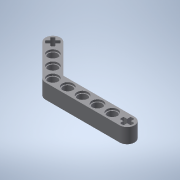
# Autodesk Inventor part: 9M Beam A 4X6
Saved by Autodesk Inventor 2021 (Build 250183000, 183)
## iProperties
Created: 2014-02-17
Part Number: 9M Beam A 4X6
Document SubType Name: Modeling
Designer: jleonard
Density: 1 g/cm^3
Material: Generic
Appearance: Default
Author: jleonard
Autodesk Inventor part; units mm, degrees
ref_plane "YZ Plane" through (0, 0, 0) normal (1, 0, 0) x (0, 1, 0)
ref_plane "XZ Plane" through (0, 0, 0) normal (0, 1, 0) x (-1, 0, 0)
ref_plane "XY Plane" through (0, 0, 0) normal (0, 0, 1) x (1, 0, 0)
sketch "Sketch1" plane through (0, 0, 0) normal (0, 0, 1) x (1, 0, 0)
  arc A0 (-54.1421, 19.799) -> (-59.799, 14.1421) centre (-56.9706, 16.9706) ccw
  arc A1 (0, -4) -> (0, 4) centre (0, 0) ccw
  line L0 (-42.8284, -2.8284) -> (-59.799, 14.1421)
  line L1 (-38.3431, 4) -> (-54.1421, 19.799)
  line L2 (-75.9529, 0) -> (17.3255, 0) projected
  line L3 (0, -9.663) -> (0, 28.0092) projected
  line L4 (0, -4) -> (-40, -4)
  line L5 (0, 4) -> (-38.3431, 4)
  arc A2 (-42.8284, -2.8284) -> (-40, -4) centre (-40, 0) ccw
  dimension "d13" = 4
  dimension "d15" = 0
  dimension "d16" = 0
  dimension "d25" = 4
  dimension "d27" = 135
  dimension "d29" = 40
  dimension "d35" = 135
  dimension "d36" = 4
  dimension "d37" = 24
  dimension "d142" = 24
  constraints: 8 end point, 6 point on circle, 4 tangent, 3 centre point, 1 parallel, 1 perpendicular, 1 point on line
  measures "d13" radius of A1
  measures "d15" distance from line of L3 A1.centre
  measures "d16" distance from line of L2 A1.centre
  measures "d25" radius of A0
  measures "d27" angle of L0 L4
  measures "d29" distance of L4.start L4.end
  measures "d35" angle of L5 L1
  measures "d36" radius of A2
  measures "d37" distance of A2.centre A0.centre
  measures "d142" distance of L0.start L0.end
extrude "Extrusion1" add sketch "Sketch1" along normal blind 8
sketch "Sketch2" plane through (0, 0, 8) normal (0, 0, 1) x (1, 0, 0)
  arc A0 (-54.1421, 19.799) -> (-59.799, 14.1421) centre (-56.9706, 16.9706) ccw projected
  line L0 (-42.8284, -2.8284) -> (-59.799, 14.1421) projected
  arc A1 (-58.2635, 19.6777) -> (-59.6777, 18.2635) centre (-56.9706, 16.9706) ccw
  arc A2 (-59.6777, 15.6777) -> (-58.2635, 14.2635) centre (-56.9706, 16.9706) ccw
  arc A3 (-55.6777, 14.2635) -> (-54.2635, 15.6777) centre (-56.9706, 16.9706) ccw
  arc A4 (-54.2635, 18.2635) -> (-55.6777, 19.6777) centre (-56.9706, 16.9706) ccw
  line L1 (-54.2635, 18.2635) -> (-55.5563, 16.9706)
  line L2 (-56.9706, 15.5563) -> (-58.2635, 14.2635)
  line L3 (-59.6777, 18.2635) -> (-58.3848, 16.9706)
  line L4 (-56.9706, 15.5563) -> (-55.6777, 14.2635)
  line L5 (-55.6777, 19.6777) -> (-56.9706, 18.3848)
  line L6 (-58.3848, 16.9706) -> (-59.6777, 15.6777)
  line L7 (-58.2635, 19.6777) -> (-56.9706, 18.3848)
  line L8 (-55.5563, 16.9706) -> (-54.2635, 15.6777)
  dimension "d46" = 3
  dimension "d47" = 3
  dimension "d48" = 3
  dimension "d49" = 3
  dimension "d50" = 2
  dimension "d51" = 2
  dimension "d52" = 2
  dimension "d53" = 2
  dimension "d54" = 1
  dimension "d55" = 1
  dimension "d56" = 1
  dimension "d57" = 1
  dimension "d58" = 90
  dimension "d59" = 90
  dimension "d60" = 90
  dimension "d61" = 90
  constraints: 16 end point, 8 point on circle, 4 centre point, 1 coincident
  measures "d46" radius of A4
  measures "d47" radius of A1
  measures "d48" radius of A2
  measures "d49" radius of A3
  measures "d50" distance between parallel lines of L6 L2
  measures "d51" distance between parallel lines of L8 L4
  measures "d52" distance between parallel lines of L5 L1
  measures "d53" distance between parallel lines of L7 L3
  measures "d54" distance from line of L3 A0.centre
  measures "d55" distance from line of L2 A0.centre
  measures "d56" distance from line of L8 A0.centre
  measures "d57" distance from line of L5 A1.centre
  measures "d58" angle of L5 L7
  measures "d59" angle of L8 L1
  measures "d60" angle of L2 L4
  measures "d61" angle of L0 L2
extrude "Extrusion2" cut sketch "Sketch2" against normal through all
sketch "Sketch3" plane through (0, 0, 8) normal (0, 0, 1) x (1, 0, 0)
  arc A0 (0, -4) -> (0, 4) centre (0, 0) ccw projected
  arc A1 (1, 2.8284) -> (-1, 2.8284) centre (0, 0) ccw
  arc A2 (-2.8284, 1) -> (-2.8284, -1) centre (0, 0) ccw
  arc A3 (-1, -2.8284) -> (1, -2.8284) centre (0, 0) ccw
  arc A4 (2.8284, -1) -> (2.8284, 1) centre (0, 0) ccw
  line L0 (-2.8284, -1) -> (-1, -1)
  line L1 (1, -1) -> (2.8284, -1)
  line L2 (-1, -2.8284) -> (-1, -1)
  line L3 (-1, 1) -> (-1, 2.8284)
  line L4 (-2.8284, 1) -> (-1, 1)
  line L5 (1, 1) -> (2.8284, 1)
  line L6 (1, -2.8284) -> (1, -1)
  line L7 (1, 1) -> (1, 2.8284)
  dimension "d65" = 3
  dimension "d66" = 3
  dimension "d67" = 3
  dimension "d68" = 3
  dimension "d69" = 2
  dimension "d70" = 2
  dimension "d71" = 2
  dimension "d72" = 2
  dimension "d73" = 90
  dimension "d74" = 90
  dimension "d75" = 90
  dimension "d76" = 1
  dimension "d77" = 1
  dimension "d78" = 1
  dimension "d79" = 1
  dimension "d80" = 2.8284
  constraints: 16 end point, 8 point on circle, 4 centre point, 1 coincident
  measures "d65" radius of A1
  measures "d66" radius of A4
  measures "d67" radius of A3
  measures "d68" radius of A2
  measures "d69" distance between parallel lines of L0 L4
  measures "d70" distance between parallel lines of L7 L3
  measures "d71" distance between parallel lines of L1 L5
  measures "d72" distance between parallel lines of L6 L2
  measures "d73" angle of L5 L7
  measures "d74" angle of L6 L1
  measures "d75" angle of L2 L0
  measures "d76" distance from line of A0.centre L3
  measures "d77" distance from line of A1.centre L0
  measures "d78" distance from line of L6 A0.centre
  measures "d79" distance from line of L5 A0.centre
  measures "d80" vertical distance of A0.centre L3.end
extrude "Extrusion3" cut sketch "Sketch3" against normal through all
sketch "Sketch10" plane through (0, 0, 8) normal (0, 0, 1) x (1, 0, 0)
  circle A0 centre (-8, 0) radius 2.5
  line L0 (-73.9647, 0) -> (16.9941, 0) projected
  line L1 (0, -21.6115) -> (0, 28.0676) projected
  circle A1 centre (-16, 0) radius 2.5
  circle A2 centre (-24, 0) radius 2.5
  circle A3 centre (-32, 0) radius 2.5
  circle A4 centre (-40, 0) radius 2.5
  point P0 (0, 0)
  dimension "d143" = 5
  dimension "d144" = 8
  dimension "d145" = 0
  dimension "d150" = 8
  constraints: 5 centre point, 1 horizontal, 8 other
  measures "d143" diameter of A0
  measures "d144" distance from line of L1 A0.centre
  measures "d145" distance from line of L0 A0.centre
  measures "d150" distance of A0.centre A1.centre
extrude "Extrusion10" cut sketch "Sketch10" against normal through all
sketch "Sketch11" plane through (0, 0, 8) normal (0, 0, 1) x (1, 0, 0)
  circle A0 centre (-45.6569, 5.6569) radius 2.5
  line L0 (-73.9647, 0) -> (16.9941, 0) projected
  line L1 (0, -8.9941) -> (0, 25.9647) projected
  line L2 (-54.1421, 19.799) -> (-38.3431, 4) projected
  circle A1 centre (-40, 0) radius 2.5 projected
  circle A2 centre (-51.3137, 11.3137) radius 2.5
  point P0 (0, 0)
  dimension "d155" = 5
  dimension "d157" = 4
  dimension "d158" = 8
  dimension "d161" = 8
  constraints: 2 centre point, 3 other
  measures "d155" diameter of A0
  measures "d157" distance from line of L2 A0.centre
  measures "d158" distance of A1.centre A0.centre
  measures "d161" distance of A0.centre A2.centre
extrude "Extrusion11" cut sketch "Sketch11" against normal through all contours A0 | A2
sketch "Sketch12" plane through (0, 0, 8) normal (0, 0, 1) x (1, 0, 0)
  circle A0 centre (-8, 0) radius 2.5 projected
  circle A1 centre (-8, 0) radius 3
  line L0 (-73.9647, 0) -> (16.9941, 0) projected
  circle A2 centre (-16, 0) radius 3
  circle A3 centre (-24, 0) radius 3
  circle A4 centre (-32, 0) radius 3
  circle A5 centre (-40, 0) radius 3
  point P0 (0, 0)
  dimension "d168" = 6
  dimension "d171" = 8
  constraints: 5 centre point, 1 coincident, 1 horizontal, 8 other
  measures "d168" diameter of A1
  measures "d171" distance of A1.centre A2.centre
extrude "Extrusion12" cut sketch "Sketch12" against normal blind 1
sketch "Sketch13" plane through (0, 0, 8) normal (0, 0, 1) x (1, 0, 0)
  circle A0 centre (-45.6569, 5.6569) radius 2.5 projected
  circle A1 centre (-51.3137, 11.3137) radius 2.5 projected
  circle A2 centre (-51.3137, 11.3137) radius 3
  circle A3 centre (-45.6569, 5.6569) radius 3
  point P0 (0, 0)
  dimension "d178" = 6
  dimension "d179" = 6
  constraints: 2 centre point, 2 coincident
  measures "d178" diameter of A2
  measures "d179" diameter of A3
extrude "Extrusion13" cut sketch "Sketch13" against normal blind 1 contours A0 | A1 | A2 | A3
sketch "Sketch14" plane through (0, 0, 0) normal (0, 0, -1) x (-1, 0, 0)
  circle A0 centre (8, 0) radius 2.5 projected
  circle A1 centre (51.3137, 11.3137) radius 2.5 projected
  circle A2 centre (45.6569, 5.6569) radius 2.5 projected
  circle A3 centre (45.6569, 5.6569) radius 3
  circle A4 centre (51.3137, 11.3137) radius 3
  circle A5 centre (8, 0) radius 3 projected
  circle A6 centre (8, 0) radius 3
  line L0 (73.9647, 0) -> (-16.9941, 0) projected
  line L1 (0, -4) -> (40, -4) projected
  circle A7 centre (16, 0) radius 3
  circle A8 centre (24, 0) radius 3
  circle A9 centre (32, 0) radius 3
  circle A10 centre (40, 0) radius 3
  point P0 (0, 0)
  dimension "d182" = 6
  dimension "d183" = 6
  dimension "d184" = 6
  dimension "d187" = 8
  constraints: 7 centre point, 3 coincident, 1 horizontal, 8 other
  measures "d182" diameter of A3
  measures "d183" diameter of A4
  measures "d184" diameter of A6
  measures "d187" distance of A6.centre A7.centre
extrude "Extrusion14" cut sketch "Sketch14" against normal blind 1 contours L0 A0 | L0 A5 A0 | A0 L0 A5 | A0 L0 | A10 L0 | L0 A10 | A9 L0 | L0 A9 | A8 L0 | L0 A8 | A7 L0 | L0 A7 | A1 | A2 | A3 | A4
body "Solid1"
